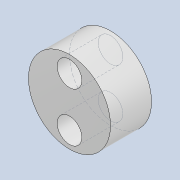
# Autodesk Inventor part: 原動節-ギア接続部
Saved by Autodesk Inventor 2020 (Build 240168000, 168)
## iProperties
Created: 2020-10-27
Part Number: 原動節-ギア接続部
Material: アルミニウム 2014-T4
Document SubType Name: Modeling
Designer: AA19065
Density: 2.8 g/cm^3
Appearance: サテン
Mass: 0.901637 g
Surface Area: 3.80133 cm^2
Volume: 0.322013 cm^3
Author: AA19065
Autodesk Inventor part; units mm, degrees
ref_plane "YZ Plane" through (0, 0, 0) normal (1, 0, 0) x (0, 1, 0)
ref_plane "XZ Plane" through (0, 0, 0) normal (0, 1, 0) x (-1, 0, 0)
ref_plane "XY Plane" through (0, 0, 0) normal (0, 0, 1) x (1, 0, 0)
sketch "スケッチ1" plane through (0, 0, 0) normal (0, 0, 1) x (1, 0, 0)
  circle A0 centre (0, 0) radius 5
  circle A1 centre (0, 3) radius 1.5
  circle A2 centre (0, -3) radius 1.5
  dimension "d0" = 10
  dimension "d1" = 3
  dimension "d6" = 3
  dimension "d11" = 360
  constraints: 3 centre point, 1 coincident, 1 vertical alignment, 5 other
  measures "d0" diameter of A0
  measures "d1" diameter of A1
  measures "d6" distance of point (0, 0) A1.centre
extrude "押し出し1" add sketch "スケッチ1" along normal blind 5
